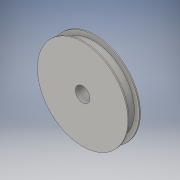
# Autodesk Inventor part: mcdave_wheel
Saved by Autodesk Inventor 2016 (Build 200138000, 138)
## iProperties
Created: 2017-09-07
Part Number: mcdave_wheel
Material: Generic
Document SubType Name: Modeling
Designer: student
Density: 1 g/cm^3
Appearance: Default
Author: student
Autodesk Inventor part; units mm, degrees
ref_plane "YZ Plane" through (0, 0, 0) normal (1, 0, 0) x (0, 1, 0)
ref_plane "XZ Plane" through (0, 0, 0) normal (0, 1, 0) x (-1, 0, 0)
ref_plane "XY Plane" through (0, 0, 0) normal (0, 0, 1) x (1, 0, 0)
sketch "Sketch1" plane through (0, 0, 0) normal (0, 0, 1) x (1, 0, 0)
  circle A0 centre (0, 0) radius 19.2532
  dimension "d0" = 38.5064
  constraints: 1 centre point, 1 coincident
  measures "d0" diameter of A0
extrude "Extrusion1" add sketch "Sketch1" along normal blind 4.9784
sketch "Sketch11" plane through (0, 0, 4.9784) normal (0, 0, 1) x (1, 0, 0)
  circle A0 centre (0, 0) radius 21.59
  dimension "d30" = 43.18
  constraints: 1 centre point, 1 coincident
  measures "d30" diameter of A0
extrude "Extrusion8" add sketch "Sketch11" along normal blind 0.508
sketch "Sketch12" plane through (0, 0, 0) normal (0, 0, -1) x (-1, 0, 0)
  circle A0 centre (0, 0) radius 21.59
  constraints: 1 centre point, 1 coincident
extrude "Extrusion9" add sketch "Sketch12" along normal blind 0.508
sketch "Sketch13" plane through (0, 0, 5.4864) normal (0, 0, 1) x (1, 0, 0)
  circle A0 centre (0, 0) radius 3.4798
  dimension "d35" = 6.9596
  constraints: 1 centre point, 1 coincident
  measures "d35" diameter of A0
extrude "Extrusion10" cut sketch "Sketch13" against normal through all
sketch "Sketch14" plane through (0, 0, -0.508) normal (0, 0, -1) x (-1, 0, 0)
  line L0 (-2.0603, -2.8043) -> (-4.6601, -5.9659)
  line L1 (-4.6601, -5.9659) -> (-2.0502, -19.1437)
  line L2 (2.0603, -2.8043) -> (4.6601, -5.9659)
  line L3 (4.6601, -5.9659) -> (2.0502, -19.1437)
  line L4 (-2.0603, 2.8043) -> (-4.6601, 5.9659)
  line L5 (-4.6601, 5.9659) -> (-2.0502, 19.1437)
  line L6 (4.6601, 5.9659) -> (2.0502, 19.1437)
  line L7 (2.0603, 2.8043) -> (4.6601, 5.9659)
  line L8 (3.3602, -0.9044) -> (6.5825, -4.3851)
  line L9 (6.5825, -4.3851) -> (19.2319, -0.9059)
  line L10 (3.3602, 0.9044) -> (6.5825, 4.3851)
  line L11 (6.5825, 4.3851) -> (19.2319, 0.9059)
  line L12 (-3.3602, -0.9044) -> (-6.5825, -4.3851)
  line L13 (-6.5825, -4.3851) -> (-19.2319, -0.9059)
  line L14 (-6.5825, 4.3851) -> (-19.2319, 0.9059)
  line L15 (-3.3602, 0.9044) -> (-6.5825, 4.3851)
  arc A0 (2.0502, 19.1437) -> (-2.0502, 19.1437) centre (0, 0) ccw
  arc A1 (-19.2319, 0.9059) -> (-19.2319, -0.9059) centre (0, 0) ccw
  arc A2 (-2.0502, -19.1437) -> (2.0502, -19.1437) centre (0, 0) ccw
  arc A3 (19.2319, -0.9059) -> (19.2319, 0.9059) centre (0, 0) ccw
  arc A4 (-2.0603, -2.8043) -> (2.0603, -2.8043) centre (0, 0) ccw
  arc A5 (-3.3602, 0.9044) -> (-3.3602, -0.9044) centre (0, 0) ccw
  arc A6 (3.3602, -0.9044) -> (3.3602, 0.9044) centre (0, 0) ccw
  arc A7 (2.0603, 2.8043) -> (-2.0603, 2.8043) centre (0, 0) ccw
  constraints: 32 end point, 16 point on circle, 8 centre point, 2 coincident
extrude "Extrusion11" add sketch "Sketch14" along normal blind 1.016
sketch "Sketch15" plane through (0, 0, -0.508) normal (0, 0, -1) x (-1, 0, 0)
  circle A0 centre (0, 0) radius 3.4798 projected
  line L0 (4.6601, -5.9659) -> (2.0502, -19.1437) projected
  line L1 (2.4217, -17.2678) -> (2.0502, -19.1437)
  constraints: 2 end point, 1 collinear, 1 point on line
body "Solid1"
